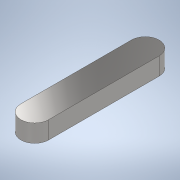
# Autodesk Inventor part: МПСТ Шпонка тихоходного вала
Saved by Autodesk Inventor 2022 (Build 260153070, 153G)
## iProperties
Created: 2021-09-23
Part Number: МПСТ Шпонка тихоходного вала
Material: Сталь, углеродистая
Document SubType Name: Modeling
Designer: Алексанян Г.
Density: 7.85 g/cm^3
Appearance: С умеренной полировкой
Author: Алексанян Г.
Autodesk Inventor part; units mm, degrees
ref_plane "YZ Plane" through (0, 0, 0) normal (1, 0, 0) x (0, 1, 0)
ref_plane "XZ Plane" through (0, 0, 0) normal (0, 1, 0) x (-1, 0, 0)
ref_plane "XY Plane" through (0, 0, 0) normal (0, 0, 1) x (1, 0, 0)
sketch "Эскиз1" plane through (0, 0, 0) normal (0, 1, 0) x (-1, 0, 0)
  line L0 (0, -44) -> (0, 44) construction
  line L1 (11, -44) -> (11, 44)
  line L2 (-11, 44) -> (-11, -44)
  arc A0 (-11, -44) -> (11, -44) centre (0, -44) ccw
  arc A1 (11, 44) -> (-11, 44) centre (0, 44) ccw
  point P0 (0, 0)
  point P1 (0, 0)
  dimension "d0" = 22
  dimension "d1" = 110
  constraints: 8 end point, 4 point on circle, 4 tangent, 2 centre point, 2 coincident, 1 midpoint, 1 parallel, 1 vertical
  measures "d0" distance between parallel lines of L2 L1
extrude "Выдавливание1" add sketch "Эскиз1" along normal blind 14
